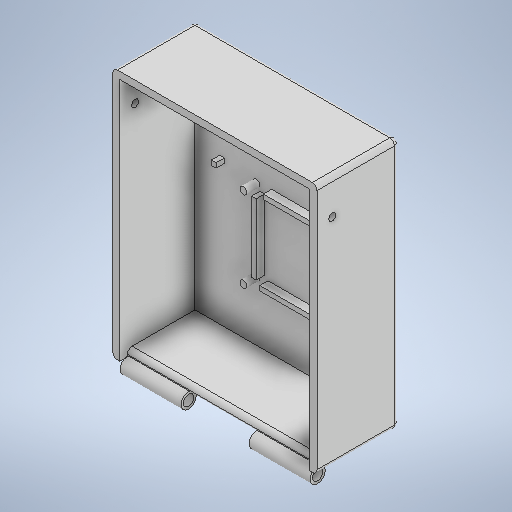
# Autodesk Inventor part: Front board
Saved by Autodesk Inventor 2025.2 (Build 292293000, 293)
## iProperties
Created: 2024-12-12
Part Number: Front board
Material: Generic
Document SubType Name: Modeling
Designer: jurre
Density: 1 g/cm^3
Appearance: Default
Author: jurre
Autodesk Inventor part; units mm, degrees
ref_plane "YZ Plane" through (0, 0, 0) normal (1, 0, 0) x (0, 1, 0)
ref_plane "XZ Plane" through (0, 0, 0) normal (0, 1, 0) x (-1, 0, 0)
ref_plane "XY Plane" through (0, 0, 0) normal (0, 0, 1) x (1, 0, 0)
sketch "Sketch2" plane through (0, 0, 0) normal (0, 0, 1) x (1, 0, 0)
  line L0 (-39.2941, 43.567) -> (41.7059, 43.567)
  line L1 (41.7059, 43.567) -> (41.7059, -57.433)
  line L2 (41.7059, -57.433) -> (-39.2941, -57.433)
  line L3 (-39.2941, -57.433) -> (-39.2941, 43.567)
  line L4 (-42.2941, 46.567) -> (44.7059, 46.567)
  line L5 (44.7059, 46.567) -> (44.7059, -60.433)
  line L6 (44.7059, -60.433) -> (-42.2941, -60.433)
  line L7 (-42.2941, -60.433) -> (-42.2941, 46.567)
  point P0 (0, 0)
  dimension "d0" = 81
  dimension "d1" = 101
  dimension "d2" = 87
  dimension "d3" = 3
  dimension "d4" = 107
  dimension "d5" = 3
  constraints: 16 end point, 4 parallel, 2 horizontal, 2 perpendicular
  measures "d0" distance of L0.start L0.end
  measures "d1" distance of L0.end L1.end
  measures "d2" distance of L4.start L4.end
  measures "d3" distance between parallel lines of L3 L7
  measures "d4" distance of L4.end L5.end
  measures "d5" distance between parallel lines of L0 L4
extrude "Extrusion1" add sketch "Sketch2" against normal blind 3 contours L0 L1 L2 L3 | L4 L5 L6 L7
extrude "Extrusion2" add sketch "Sketch2" along normal blind 32
sketch "Sketch4" plane through (-42.2941, -60.433, -3) normal (-1, 0, 0) x (0, 0, 1)
  line L0 (35, 0) -> (0, 0) projected
  line L1 (35, 107) -> (35, 0) projected
  circle A0 centre (31.7351, -3) radius 3.25
  circle A1 centre (31.7351, -3) radius 2.25
  circle A2 centre (31.7351, -3) radius 2
  point P0 (3, 60.433)
  point P1 (32.9851, 0)
  point P2 (30.4851, 0)
  dimension "d13" = 3
  dimension "d14" = 6.5
  dimension "d15" = 3.2649
  dimension "d16" = 4.5
  dimension "d17" = 4
  constraints: 3 centre point, 2 coincident
  measures "d13" distance from line of L0 A0.centre
  measures "d14" diameter of A0
  measures "d15" distance from line of A0.centre L1
  measures "d16" diameter of A1
  measures "d17" diameter of A2
extrude "Extrusion3" add sketch "Sketch4" against normal blind 26 separate body contours A0 L0 | L0 A0
move or copy body "Move Body1" bodies to move or copy 2 copy no translate (58, 0, 0)
extrude "Extrusion4" add sketch "Sketch4" against normal blind 26 separate body contours A0 L0 | L0 A0
sketch "Sketch5" plane through (-39.2941, -57.433, 0) normal (0, 1, 0) x (1, 0, 0)
  line L0 (81, -32) -> (0, -32) projected
  line L1 (81, 0) -> (81, -32) projected
  line L2 (0, -32) -> (81, -32)
  line L3 (81, -32) -> (81, -28.8)
  line L4 (81, -28.8) -> (0, -28.8)
  line L5 (0, -28.8) -> (0, -32)
  point P0 (39.2941, 0)
  dimension "d138" = 3.2
  constraints: 8 end point, 2 parallel, 1 horizontal, 1 perpendicular, 1 point on line
  measures "d138" distance between parallel lines of L0 L4
extrude "Extrusion5" cut sketch "Sketch5" against normal blind 29 bodies 1
sketch "Sketch6" plane through (0, 0, 0) normal (0, 0, 1) x (1, 0, 0)
  line L0 (31.2059, 4.873) -> (-28.7941, 4.873)
  line L1 (-28.7941, 4.873) -> (-28.7941, -34.627)
  line L2 (-28.7941, -34.627) -> (31.2059, -34.627)
  line L3 (31.2059, -34.627) -> (31.2059, 4.873)
  line L4 (-11.6723, -29.877) -> (-9.6723, -29.877)
  line L5 (-9.6723, -29.877) -> (-9.6723, 0.123)
  line L6 (-9.6723, 0.123) -> (-11.6723, 0.123)
  line L7 (-11.6723, 0.123) -> (-11.6723, -29.877)
  line L8 (29.7059, 0.123) -> (27.7059, 0.123)
  line L9 (27.7059, 0.123) -> (27.7059, -29.777)
  line L10 (27.7059, -29.777) -> (29.7059, -29.777)
  line L11 (29.7059, -29.777) -> (29.7059, 0.123)
  circle A0 centre (24.6059, -28.027) radius 1.5
  circle A1 centre (24.6059, -1.727) radius 1.5
  circle A2 centre (-13.1723, -32.127) radius 1.5
  circle A3 centre (-13.1723, 2.373) radius 1.5
  line L12 (-6.6723, 3.373) -> (23.3277, 3.373)
  line L13 (23.3277, 3.373) -> (23.3277, 1.373)
  line L14 (23.3277, 1.373) -> (-6.6723, 1.373)
  line L15 (-6.6723, 1.373) -> (-6.6723, 3.373)
  line L16 (-8.1723, -31.127) -> (21.8277, -31.127)
  line L17 (21.8277, -31.127) -> (21.8277, -33.127)
  line L18 (21.8277, -33.127) -> (-8.1723, -33.127)
  line L19 (-8.1723, -33.127) -> (-8.1723, -31.127)
  line L20 (-28.7941, 4.873) -> (-26.7941, 4.873)
  line L21 (-26.7941, 4.873) -> (-26.7941, 2.873)
  line L22 (-26.7941, 2.873) -> (-28.7941, 2.873)
  line L23 (-28.7941, 2.873) -> (-28.7941, 4.873)
  line L24 (-39.2941, -60.433) -> (-39.2941, 43.567) projected
  line L25 (41.7059, 43.567) -> (41.7059, -60.433) projected
  point P0 (0, 0)
  point P1 (21.8292, -7.4376)
  point P2 (-8.1723, -32.127)
  point P3 (-31.4705, 14.6914)
  point P4 (-29.4705, 16.6914)
  point P5 (-26.7941, 4.873)
  dimension "d27" = 60
  dimension "d28" = 39.5
  dimension "d29" = 2
  dimension "d30" = 4.75
  dimension "d31" = 2
  dimension "d32" = 1.5
  dimension "d33" = 4.75
  dimension "d34" = 4.85
  dimension "d35" = 3
  dimension "d36" = 6.6
  dimension "d37" = 6.6
  dimension "d38" = 3
  dimension "d39" = 6.6
  dimension "d40" = 6.6
  dimension "d41" = 3
  dimension "d42" = 2.5
  dimension "d43" = 3
  dimension "d44" = 2.5
  dimension "d45" = 35
  dimension "d46" = 1.5
  dimension "d47" = 35
  dimension "d48" = 1.5
  dimension "d49" = 30
  dimension "d50" = 5
  dimension "d51" = 2
  dimension "d52" = 5
  dimension "d53" = 1.5
  dimension "d54" = 30
  dimension "d55" = 2
  dimension "d56" = 2
  dimension "d57" = 2
  dimension "d68" = 10.5
  dimension "d69" = 10.5
  constraints: 48 end point, 12 parallel, 6 horizontal, 6 perpendicular, 4 centre point, 1 midpoint
  measures "d27" distance of L2.end L1.end
  measures "d28" distance of L1.end L0.end
  measures "d29" distance of L6.end L5.end
  measures "d30" distance between parallel lines of L0 L6
  measures "d31" distance of L10.end L9.end
  measures "d32" distance between parallel lines of L3 L11
  measures "d33" distance between parallel lines of L0 L8
  measures "d34" distance between parallel lines of L2 L10
  measures "d35" diameter of A0
  measures "d36" distance from line of L2 A0.centre
  measures "d37" distance from line of L3 A0.centre
  measures "d38" diameter of A1
  measures "d39" distance from line of L0 A1.centre
  measures "d40" distance from line of L3 A1.centre
  measures "d41" diameter of A2
  measures "d42" distance from line of L2 A2.centre
  measures "d43" diameter of A3
  measures "d44" distance from line of L0 A3.centre
  measures "d46" distance from line of L7 A2.centre
  measures "d48" distance between parallel lines of L2 L18
  measures "d49" distance of L16.start L16.end
  measures "d50" distance of A2.centre point (-8.172, -32.127)
  measures "d51" distance of L16.end L17.end
  measures "d52" distance edge to line of A3 L15
  measures "d53" distance between parallel lines of L0 L12
  measures "d54" distance of L13.end L14.end
  measures "d55" distance of L12.end L13.end
  measures "d56" distance of L21.end L22.end
  measures "d57" distance of L20.end L21.end
  measures "d68" distance between parallel lines of L24 L1
  measures "d69" distance between parallel lines of L25 L3
sketch "Sketch7" plane through (0, 0, 0) normal (0, 0, 1) x (1, 0, 0)
  circle A0 centre (1.2059, 28.567) radius 2.5
  line L0 (-39.2941, 43.567) -> (41.7059, 43.567) projected
  line L1 (41.7059, 43.567) -> (41.7059, -60.433) projected
  line L2 (-39.2941, -60.433) -> (-39.2941, 43.567) projected
  point P0 (0, 0)
  dimension "d63" = 5
  dimension "d64" = 15
  dimension "d65" = 81
  dimension "d66" = 40.5
  dimension "d67" = 40.5
  constraints: 1 centre point
  measures "d63" diameter of A0
  measures "d64" distance from line of L0 A0.centre
  measures "d65" distance between parallel lines of L1 L2
  measures "d66" distance from line of L1 A0.centre
  measures "d67" distance from line of L2 A0.centre
extrude "Extrusion8" cut sketch "Sketch7" against normal blind 5.5 bodies 1
extrude "Extrusion9" add sketch "Sketch6" along normal blind 5.5 contours A0 | A1 | A2 | A3 bodies 1
extrude "Extrusion10" add sketch "Sketch6" along normal blind 3.5 contours L21 L22 L1 L0 | L7 L6 L5 L4 | L11 L10 L9 L8 | L12 L13 L14 L15 | L16 L17 L18 L19 bodies 1
fillet "Fillet2" radius 1 1 edges at (-1.2941, 28.567, -3)
sketch "Sketch8" plane through (0, 0, -3) normal (0, 0, -1) x (-1, 0, 0)
  line L0 (-44.7059, 43.567) -> (-44.7059, -57.433) projected
  line L1 (42.2941, -57.433) -> (42.2941, 43.567) projected
  line L2 (-41.7059, -60.433) -> (39.2941, -60.433) projected
  line L3 (-33.7059, 8.8111) -> (30.2941, 8.8111)
  line L4 (32.2941, 6.8111) -> (32.2941, -40.7857)
  line L5 (30.2941, -42.7857) -> (-33.7059, -42.7857)
  line L6 (-35.7059, -40.7857) -> (-35.7059, 6.8111)
  arc A0 (-33.7059, 8.8111) -> (-35.7059, 6.8111) centre (-33.7059, 6.8111) ccw
  arc A1 (32.2941, 6.8111) -> (30.2941, 8.8111) centre (30.2941, 6.8111) ccw
  arc A2 (30.2941, -42.7857) -> (32.2941, -40.7857) centre (30.2941, -40.7857) ccw
  arc A3 (-35.7059, -40.7857) -> (-33.7059, -42.7857) centre (-33.7059, -40.7857) ccw
  line L7 (-33.7059, 9.8111) -> (30.2941, 9.8111)
  line L8 (33.2941, 6.8111) -> (33.2941, -40.7857)
  line L9 (30.2941, -43.7857) -> (-33.7059, -43.7857)
  line L10 (-36.7059, -40.7857) -> (-36.7059, 6.8111)
  arc A4 (-33.7059, 9.8111) -> (-36.7059, 6.8111) centre (-33.7059, 6.8111) ccw
  arc A5 (33.2941, 6.8111) -> (30.2941, 9.8111) centre (30.2941, 6.8111) ccw
  arc A6 (30.2941, -43.7857) -> (33.2941, -40.7857) centre (30.2941, -40.7857) ccw
  arc A7 (-36.7059, -40.7857) -> (-33.7059, -43.7857) centre (-33.7059, -40.7857) ccw
  arc A8 (-6.6412, -12.6618) -> (-6.2337, -20.9909) centre (-0.99, -16.5599) ccw
  arc A9 (-8.5878, -11.3347) -> (-8.1085, -22.4256) centre (-1.4098, -16.5802) ccw
  arc A10 (-6.5691, -12.2512) -> (-8.2567, -11.135) centre (-8.0364, -12.6357) ccw
  arc A11 (-7.9843, -22.5283) -> (-6.1239, -21.223) centre (-7.353, -21.4496) ccw
  arc A12 (-10.22, -10.3231) -> (-9.8927, -23.0813) centre (-1.8137, -16.4908) ccw
  arc A13 (-12.013, -9.2144) -> (-11.8184, -24.7342) centre (-2.6986, -16.8587) ccw
  arc A14 (-10.139, -9.9025) -> (-11.8214, -9.0711) centre (-11.3385, -10.2119) ccw
  arc A15 (-11.663, -24.8549) -> (-9.8062, -23.2379) centre (-11.0688, -23.6627) ccw
  arc A16 (-13.6116, -8.3071) -> (-13.5954, -25.7887) centre (-2.8343, -17.0379) ccw
  arc A17 (-15.3535, -6.9426) -> (-15.4491, -27.1869) centre (-2.9826, -17.1234) ccw
  arc A18 (-13.5172, -8.1218) -> (-15.2232, -6.8307) centre (-14.6325, -7.8228) ccw
  arc A19 (-15.3878, -27.2505) -> (-13.5197, -25.9168) centre (-14.6141, -26.359) ccw
  arc A20 (-17.4362, -5.8537) -> (-17.4341, -28.0943) centre (-3.3787, -16.9727) ccw
  arc A21 (-19.0576, -4.549) -> (-19.0185, -29.3675) centre (-5.356, -16.9367) ccw
  arc A22 (-17.3386, -5.6445) -> (-18.9107, -4.4372) centre (-18.4174, -5.422) ccw
  arc A23 (-18.9817, -29.404) -> (-17.3782, -28.1826) centre (-18.298, -28.6383) ccw
  arc A24 (4.4596, -21.376) -> (3.9921, -12.9185) centre (-2.1078, -17.4973) ccw
  arc A25 (6.2852, -22.4425) -> (5.7436, -11.6396) centre (-0.7047, -17.3779) ccw
  arc A26 (4.3941, -21.5678) -> (6.2141, -22.5215) centre (5.4821, -21.7048) ccw
  arc A27 (5.6288, -11.5441) -> (3.8969, -12.6885) centre (5.0344, -12.5272) ccw
  arc A28 (8.0044, -23.3696) -> (7.6623, -10.6806) centre (-0.5228, -17.2503) ccw
  arc A29 (9.8406, -24.6255) -> (9.2564, -9.3436) centre (-0.0541, -17.3516) ccw
  arc A30 (9.0655, -9.2064) -> (7.5642, -10.4764) centre (8.6478, -10.2349) ccw
  arc A31 (7.9006, -23.5864) -> (9.7533, -24.7172) centre (9.0269, -23.8242) ccw
  arc A32 (11.2511, -25.6135) -> (11.2437, -8.0739) centre (-0.2069, -16.8485) ccw
  arc A33 (13.0257, -27.1157) -> (13.1592, -6.9118) centre (0.6406, -16.9314) ccw
  arc A34 (13.1592, -6.9118) -> (11.1533, -7.8817) centre (12.267, -7.6259) ccw
  arc A35 (11.1563, -25.8275) -> (12.7866, -27.276) centre (12.4113, -26.0567) ccw
  arc A36 (15.0895, -28.058) -> (15.13, -6.0187) centre (0.5125, -17.0116) ccw
  arc A37 (16.9774, -29.204) -> (17.0267, -4.7249) centre (1.4905, -16.9333) ccw
  arc A38 (17.0267, -4.7249) -> (15.078, -5.9329) centre (16.1197, -5.4376) ccw
  arc A39 (15.0017, -28.2436) -> (16.9774, -29.204) centre (16.0957, -28.5054) ccw
  arc A40 (3.8969, -12.6885) -> (3.9921, -12.9185) centre (4.392, -12.6183) ccw
  arc A41 (5.7436, -11.6396) -> (5.6288, -11.5441) centre (5.3701, -11.972) ccw
  arc A42 (9.2564, -9.3436) -> (9.0655, -9.2064) centre (8.8774, -9.6696) ccw
  arc A43 (7.5642, -10.4764) -> (7.6623, -10.6806) centre (8.0522, -10.3676) ccw
  arc A44 (11.1533, -7.8817) -> (11.2437, -8.0739) centre (11.6406, -7.7698) ccw
  arc A45 (13.1592, -6.9118) -> (13.1592, -6.9118) centre (13.5496, -6.5994) ccw
  arc A46 (15.078, -5.9329) -> (15.13, -6.0187) centre (15.5296, -5.7182) ccw
  arc A47 (17.0267, -4.7249) -> (17.0267, -4.7249) centre (17.4199, -4.416) ccw
  arc A48 (16.9774, -29.204) -> (16.9774, -29.204) centre (17.3693, -29.5145) ccw
  arc A49 (15.0895, -28.058) -> (15.0017, -28.2436) centre (15.488, -28.36) ccw
  arc A50 (12.7866, -27.276) -> (13.0257, -27.1157) centre (12.6395, -26.7981) ccw
  arc A51 (11.2511, -25.6135) -> (11.1563, -25.8275) centre (11.6482, -25.9173) ccw
  arc A52 (9.7533, -24.7172) -> (9.8406, -24.6255) centre (9.4378, -24.3293) ccw
  line L11 (7.9853, -23.3958) -> (8.0044, -23.3696)
  arc A53 (7.9853, -23.3958) -> (7.9006, -23.5864) centre (8.3898, -23.6897) ccw
  arc A54 (4.4596, -21.376) -> (4.3941, -21.5678) centre (4.8901, -21.6303) ccw
  arc A55 (6.2141, -22.5215) -> (6.2852, -22.4425) centre (5.8803, -22.1492) ccw
  arc A56 (-6.1239, -21.223) -> (-6.2337, -20.9909) centre (-6.6156, -21.3136) ccw
  arc A57 (-8.1085, -22.4256) -> (-7.9843, -22.5283) centre (-7.7317, -22.0968) ccw
  arc A58 (-6.6412, -12.6618) -> (-6.5691, -12.2512) centre (-7.0528, -12.3779) ccw
  arc A59 (-8.2567, -11.135) -> (-8.5878, -11.3347) centre (-8.1841, -11.6297) ccw
  arc A60 (-10.22, -10.3231) -> (-10.139, -9.9025) centre (-10.6231, -10.0274) ccw
  arc A61 (-11.8214, -9.0711) -> (-12.013, -9.2144) centre (-11.6265, -9.5316) ccw
  arc A62 (-11.8184, -24.7342) -> (-11.663, -24.8549) centre (-11.44, -24.4074) ccw
  arc A63 (-9.8062, -23.2379) -> (-9.8927, -23.0813) centre (-10.2801, -23.3974) ccw
  arc A64 (-13.5197, -25.9168) -> (-13.5954, -25.7887) centre (-13.9833, -26.1041) ccw
  arc A65 (-15.4491, -27.1869) -> (-15.3878, -27.2505) centre (-15.0601, -26.8729) ccw
  arc A66 (-17.3782, -28.1826) -> (-17.4341, -28.0943) centre (-17.8262, -28.4046) ccw
  arc A67 (-19.0185, -29.3675) -> (-18.9817, -29.404) centre (-18.6487, -29.0311) ccw
  arc A68 (-17.4362, -5.8537) -> (-17.3386, -5.6445) centre (-17.8283, -5.5435) ccw
  arc A69 (-18.9107, -4.4372) -> (-19.0576, -4.549) centre (-18.6868, -4.8843) ccw
  arc A70 (-15.2232, -6.8307) -> (-15.3535, -6.9426) centre (-14.9674, -7.2603) ccw
  arc A71 (-13.6116, -8.3071) -> (-13.5172, -8.1218) centre (-14.0001, -7.9923) ccw
  point P0 (0, 0)
  point P1 (7.9318, -23.4695)
  point P2 (13.1592, -6.9118)
  point P3 (16.9774, -29.204)
  point P4 (17.0267, -4.7249)
  dimension "d113" = 2
  dimension "d117" = 1
  dimension "d119" = 1
  dimension "d120" = 1
  dimension "d121" = 1
  dimension "d123" = 3
  dimension "d127" = 0.5
  dimension "d128" = 0.5
  dimension "d130" = 0.5
  constraints: 146 point on circle, 83 tangent, 72 centre point, 34 equal radius, 18 end point, 4 parallel, 2 horizontal, 2 perpendicular, 1 point on line
  measures "d113" radius of A0
  measures "d117" distance between parallel lines of L7 L3
  measures "d119" distance between parallel lines of L4 L8
  measures "d120" distance between parallel lines of L5 L9
  measures "d121" distance between parallel lines of L6 L10
  measures "d123" radius of A4
  measures "d127" radius of A40
  measures "d128" radius of A44
  measures "d130" radius of A54
extrude "Extrusion13" cut sketch "Sketch8" against normal blind 0.3 contours L7 A5 L8 A6 L9 A7 L10 A4 | A8 A56 A11 A57 A9 A59 A10 A58 | A12 A63 A15 A62 A13 A61 A14 A60 | A16 A64 A19 A65 A17 A70 A18 A71 | A20 A66 A23 A67 A21 A69 A22 A68 | A24 A40 A27 A41 A25 A55 A26 A54 | A28 A43 A30 A42 A29 A52 A31 A53 L11 | A32 A44 A34 A33 A50 A35 A51 | A36 A46 A38 A37 A39 A49 bodies 1
fillet "Fillet3" radius 0.1 78 edges at (35.8272, 8.9325, -3) (1.7059, 9.8111, -3) (-32.4154, 8.9325, -3) (-33.2941, -16.9873, -3) (-32.4154, -42.9071, -3) (1.7059, -43.7857, -3) (35.8272, -42.9071, -3) (36.7059, -16.9873, -3) (35.1201, -42.2, -3) (1.7059, -42.7857, -3) (-31.7083, -42.2, -3) (-32.2941, -16.9873, -3) (-31.7083, 8.2253, -3) (1.7059, 8.8111, -3) (35.1201, 8.2253, -3) (35.7059, -16.9873, -3) (18.9894, -4.4863, -3) (17.7465, -4.5485, -3) (17.3752, -5.7548, -3) (21.302, -16.9744, -3) (17.4038, -28.137, -3) (17.676, -29.4549, -3) (19.0006, -29.3863, -3) (23.8273, -16.9658, -3) (15.2932, -6.881, -3) (13.9356, -6.9021, -3) (13.5547, -8.2194, -3) (16.7043, -17.0508, -3) (13.5527, -25.8499, -3) (13.9283, -27.3197, -3) (15.4199, -27.2201, -3) (19.0039, -17.0477, -3) (9.8424, -23.1557, -3) (10.194, -24.6673, -3) (11.7467, -24.8023, -3) (14.7473, -17.0098, -3) (11.9259, -9.1311, -3) (10.7897, -9.1013, -3) (10.1321, -10.1219, -3) (12.2365, -16.7582, -3) (6.1636, -21.0998, -3) (6.6351, -22.4727, -3) (8.0505, -22.482, -3) (10.2919, -16.9641, -3) (8.4423, -11.2015, -3) (7.1996, -11.3706, -3) (6.5603, -12.4644, -3) (7.847, -16.8953, -3) (-3.93, -12.8095, -3) (-4.401, -11.5687, -3) (-5.6898, -11.5875, -3) (-7.9164, -16.9457, -3) (-6.2518, -22.4839, -3) (-4.9731, -22.6762, -3) (-4.417, -21.4685, -3) (-5.5078, -17.0764, -3) (-9.7999, -24.6741, -3) (-8.4272, -24.8068, -3) (-7.9329, -23.4867, -3) (-7.9948, -23.3827, -3) (-9.1692, -9.2636, -3) (-7.9308, -9.3873, -3) (-7.6015, -10.5841, -3) (-9.969, -16.9675, -3) (-12.2176, -16.8825, -3) (-12.9179, -27.2134, -3) (-11.564, -27.0103, -3) (-11.191, -25.7149, -3) (-14.2191, -16.8425, -3) (-11.1882, -7.9826, -3) (-11.7696, -6.5971, -3) (-16.6749, -17.0374, -3) (-15.604, -29.5171, -3) (-15.0359, -28.1463, -3) (-18.8021, -17.0452, -3) (-15.1018, -5.9771, -3) (-15.512, -4.4572, -3) (-21.2494, -16.973, -3)
move or copy body "Move Body2" bodies to move or copy 3 copy no translate (3, 0, 0)
fillet "Fillet4" radius 2 9 edges at (1.2059, -57.433, 28.8) (44.7059, 46.567, 14.5) (1.2059, 46.567, -3) (44.7059, -6.933, -3) (-42.2941, 46.567, 14.5) (44.7059, -60.433, 14.5) (1.2059, -60.433, -3) (-42.2941, -6.933, -3) (-42.2941, -60.433, 14.5)
fillet "Fillet5" radius 1 1 edges at (1.2059, -60.433, 28.8)
sketch "Sketch9" plane through (-39.2941, -60.433, 32) normal (1, 0, 0) x (0, 0, -1)
  circle A0 centre (6.5, 92) radius 1.5
  line L0 (32, 104) -> (0, 104) projected
  line L1 (0, 2) -> (0, 105) projected
  point P0 (32, 60.433)
  dimension "d144" = 3
  dimension "d145" = 12
  dimension "d148" = 6.5
  constraints: 1 centre point
  measures "d144" diameter of A0
  measures "d145" distance from line of L0 A0.centre
  measures "d148" distance from line of L1 A0.centre
extrude "Extrusion14" cut sketch "Sketch9" along normal mid plane 200 bodies 1
combine bodies "Combine2" operation type add bodies to combine 1 3 2
body "Solid1"
